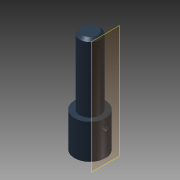
# Autodesk Inventor part: 13_0204_062
Saved by Autodesk Inventor 2012 SP1 (Build 160190100, 190)
## iProperties
Created: 2013-04-29
Part Number: 13_0204_062
Material: Default
Document SubType Name: Modeling
Designer: vogel
Density: 1 g/cm^3
Author: vogel
Autodesk Inventor part; units mm, degrees
note: some values were not read from the file. Chosen so that the rebuilt part matches the saved one: direction of "Bohrung2".
ref_plane "XZ Plane" through (0, 0, 0) normal (0, 1, 0) x (-1, 0, 0)
ref_plane "XY Plane" through (0, 0, 0) normal (0, 0, 1) x (1, 0, 0)
sketch "Skizze1" plane through (0, 0, 0) normal (0, 0, 1) x (1, 0, 0)
  circle A0 centre (0, 0) radius 6
  dimension "d0" = 12
  constraints: 1 centre point, 1 coincident
  measures "d0" diameter of A0
extrude "Extrusion1" add sketch "Skizze1" along normal blind 13.5
sketch "Skizze2" plane through (0, 0, 13.5) normal (0, 0, 1) x (1, 0, 0)
  circle A0 centre (0, 0) radius 6 projected
  circle A1 centre (0, 0) radius 4
  dimension "d3" = 8
  constraints: 1 centre point, 1 coincident
  measures "d3" diameter of A1
extrude "Extrusion2" add sketch "Skizze2" along normal blind 26.5 contours A1
sketch "Skizze3" plane through (0, 0, 0) normal (0, 0, -1) x (-1, 0, 0)
  circle A0 centre (0, 0) radius 6 projected
  constraints: 1 coincident
hole "Bohrung1" at (0, 0, 0) direction (0, 0, 1) diameter 5 depth 25 tip angle 118
ref_plane "Arbeitsebene1" through (6, 0, 0) normal (1, 0, 0) x (0, 1, 0)
sketch "Skizze4" plane through (6, 0, 0) normal (1, 0, 0) x (0, 1, 0)
  line L0 (-8.4, 0) -> (8.4, 0) projected
  line L1 (0, -2.7) -> (0, 16.2) projected
  point P0 (0, 0)
  point P1 (0, 10)
  dimension "d13" = 10
  constraints: 1 point on line
  measures "d13" distance from line of L0 point (0, 10)
hole "Bohrung2" at (6, 0, 10) direction (-1, 0, 0) diameter 2.459 end up to surface thread size "M3x0.5" class "6H" standard "ISO Metric profile"
chamfer "Fase1" distance 1 angle 45 1 edges at (-4, 0, 40)
